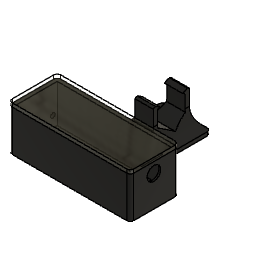
Sun_Flower_Step_Up_Support (Autodesk Fusion 360 design; units mm, degrees)
Autodesk Fusion 360 part; units mm, degrees
sketch "Sketch1" plane through (0, 0, 0) normal (0, 0, 1) x (1, 0, 0)
  line L0 (25, 9) -> (-25, 9)
  line L1 (-25, 9) -> (-25, -9)
  line L2 (-25, -9) -> (25, -9)
  line L3 (25, -9) -> (25, 9)
  line L4 (25, 9) -> (-25, -9) construction
  line L5 (-25, 9) -> (25, -9) construction
  line L6 (-26.6, -10.6) -> (26.6, -10.6)
  line L7 (26.6, -10.6) -> (26.6, 10.6)
  line L8 (26.6, 10.6) -> (-26.6, 10.6)
  line L9 (-26.6, 10.6) -> (-26.6, -10.6)
  dimension "d1" = 50
  dimension "d2" = 18
  dimension "d5" = 1.6
  constraint horizontal L0
  constraint perpendicular L0 L1
  constraint parallel L0 L2
  constraint parallel L1 L3
  constraint coincident L4 origin
  constraint coincident L5 origin
  measures "d1" distance of L1.end L2.end
  measures "d2" distance of L0.end L1.end
extrude "Extrude1" add sketch "Sketch1" along normal blind 1.2 contours L0 L1 L2 L3 makes body 1
extrude "Extrude2" add sketch "Sketch1" along normal blind 18 bodies 1
sketch "Sketch6" plane through (25, 0, 0) normal (-1, 0, 0) x (0, -1, 0)
  line L0 (-9, 1.2) -> (9, 1.2)
  line L1 (9, 1.2) -> (9, 18)
  line L2 (9, 18) -> (-9, 18)
  line L3 (-9, 18) -> (-9, 1.2)
  line L4 (-4.3225, 18) -> (4.8375, 18)
  line L5 (4.8375, 18) -> (4.8375, 6.4)
  line L6 (4.8375, 6.4) -> (-4.3225, 6.4)
  line L7 (-4.3225, 6.4) -> (-4.3225, 18)
  line L8 (4.6375, 6.6) -> (-4.1225, 6.6)
  line L9 (-4.1225, 6.6) -> (-4.1225, 17.8)
  line L10 (-4.1225, 17.8) -> (4.6375, 17.8)
  line L11 (4.6375, 17.8) -> (4.6375, 6.6)
  point P0 (-4.3225, 18)
  point P1 (4.8375, 6.4)
  dimension "d27" = 0.2
  dimension "d62" = 11.6
  constraint horizontal L4
  constraint vertical L5
  constraint horizontal L6
  constraint vertical L7
  constraint coincident P1 L5.end
  constraint coincident P0 L4.start
  constraint coincident L2 L4.end
  measures "d62" distance of L4 L6
extrude "Extrude3" cut sketch "Sketch6" against normal blind 0.8 contours L2 L4 L5 L6 L7 | L8 L9 L10 L11 bodies 1
sketch "Sketch3" plane through (26.6, 0, 0) normal (1, 0, 0) x (0, 1, 0)
  line L0 (-10.6, 0) -> (10.6, 0)
  line L1 (10.6, 0) -> (10.6, 18)
  line L2 (10.6, 18) -> (-10.6, 18)
  line L3 (-10.6, 18) -> (-10.6, 0)
  circle A0 centre (-0.2575, 13.52) radius 3
  dimension "d63" = 4.48
  measures "d63" distance of L2 A0.centre
extrude "Extrude4" cut sketch "Sketch3" against normal blind 2 contours A0 bodies 1
sketch "Sketch4" plane through (-26.6, 0, 0) normal (-1, 0, 0) x (0, -1, 0)
  line L0 (-10.6, 0) -> (10.6, 0)
  line L1 (10.6, 0) -> (10.6, 18)
  line L2 (10.6, 18) -> (-10.6, 18)
  line L3 (-10.6, 18) -> (-10.6, 0)
  circle A0 centre (-7.1, 6) radius 1
  dimension "d13" = 2
  dimension "d14" = 6
  dimension "d15" = 3.5
  measures "d13" diameter of A0
  measures "d14" distance of L0 A0.centre
  measures "d15" distance of L3 A0.centre
extrude "Extrude5" cut sketch "Sketch4" against normal blind 1.6 contours A0 bodies 1
mirror "Mirror1" about plane through (0, 0, 0) normal (0, 1, 0) of "Extrude5"
sketch "Sketch5" plane through (0, 0, 18) normal (0, 0, 1) x (-1, 0, 0)
  line L0 (26.6, -10.6) -> (26.6, 10.6)
  line L1 (26.6, 10.6) -> (-26.6, 10.6)
  line L2 (-26.6, 10.6) -> (-26.6, -10.6)
  line L3 (-26.6, -10.6) -> (26.6, -10.6)
  line L4 (-25, 4.8375) -> (-25, 9)
  line L5 (-25, 9) -> (25, 9)
  line L6 (25, 9) -> (25, -9)
  line L7 (25, -9) -> (-25, -9)
  line L8 (26.6, -10.6) -> (-26.6, -10.6)
  line L9 (-26.6, -10.6) -> (-26.6, 10.6)
  line L10 (-26.6, 10.6) -> (26.6, 10.6)
  line L11 (26.6, 10.6) -> (26.6, -10.6)
  line L12 (-25.8, -4.3225) -> (-25.8, 4.8375)
  line L13 (-25.8, 4.8375) -> (-25, 4.8375)
  line L14 (-25, -9) -> (-25, -4.3225)
  line L15 (-25, -4.3225) -> (-25.8, -4.3225)
  line L16 (26.6, -10.6) -> (26.6, 10.6)
  line L17 (26.6, 10.6) -> (-26.6, 10.6)
  line L18 (-26.6, 10.6) -> (-26.6, -10.6)
  line L19 (-26.6, -10.6) -> (26.6, -10.6)
  line L20 (-25, -4.3225) -> (-25.8, -4.3225)
  line L21 (-25.8, -4.3225) -> (-25.8, 4.8375)
  line L22 (-25.8, 4.8375) -> (-25, 4.8375)
  line L23 (-25, 4.8375) -> (-25, 9)
  line L24 (-25, 9) -> (25, 9)
  line L25 (25, 9) -> (25, -9)
  line L26 (25, -9) -> (-25, -9)
  line L27 (-25, -9) -> (-25, -4.3225)
  constraint horizontal L8
  constraint vertical L9
  constraint horizontal L10
  constraint vertical L11
  constraint coincident L1.end L2.start
  constraint coincident L0.start L3.end
extrude "Extrude7" add sketch "Sketch5" along normal blind 1.6 separate body contours L0 L1 L2 L3 L8 L9 L10 L11 L16 L17 L18 L19 | L4 L5 L6 L7 L12 L13 L14 L15 L20 L21 L22 L23 L24 L25 L26 L27 makes body 2
fillet "Fillet1" radius 1.5 8 edges at (-26.6, -10.6, 9) (-26.6, 10.6, 9) (26.6, 10.6, 9) (26.6, -10.6, 9) (-26.6, -10.6, 18.8) (-26.6, 10.6, 18.8) (26.6, 10.6, 18.8) (26.6, -10.6, 18.8) on bodies 1 2
move_body "Move4" bodies 2 to x (1, 0, 0) y (0, 1, 0) z (0, 0, 1) at (0, 0, -0.15)
sketch "Sketch9" plane through (0, 0, 1.2) normal (0, 0, 1) x (-1, 0, 0)
  line L0 (-25, 9) -> (-25, -9)
  line L1 (-25, -9) -> (25, -9)
  line L2 (25, -9) -> (25, 9)
  line L3 (25, 9) -> (-25, 9)
  circle A0 centre (23.5, 7.15) radius 1
  circle A1 centre (-10, 7.15) radius 1
  dimension "d49" = 2
  dimension "d50" = 1.5
  dimension "d51" = 1.85
  dimension "d56" = 2
  dimension "d57" = 15
  dimension "d58" = 1.85
  measures "d49" diameter of A0
  measures "d50" distance of L2 A0.centre
  measures "d51" distance of L3 A0.centre
  measures "d56" diameter of A1
  measures "d57" distance of L0 A1.centre
  measures "d58" distance of L3 A1.centre
extrude "Extrude12" cut sketch "Sketch9" against normal blind 1.2 contours A0 | A1 bodies 1
mirror "Mirror2" about plane through (0, 0, 0) normal (0, 1, 0) of "Extrude12"
move_body "Move1" bodies 2 to x (1, 0, 0) y (0, 1, 0) z (0, 0, 1) at (0, 0, 0.0101)
move_body "Move5" bodies 2 to x (1, 0, 0) y (0, 1, 0) z (0, 0, 1) at (0, 0, 0.15)
sketch "Sketch7" plane through (0, 0, 0) normal (0, 0, 1) x (1, 0, 0)
  line L0 (10.6, -10.6) -> (-10.6, -10.6)
  line L1 (-10.6, -10.6) -> (-10.6, 10.6)
  line L2 (-10.6, 10.6) -> (10.6, 10.6)
  line L3 (10.6, 10.6) -> (10.6, -10.6)
  line L4 (10.6, -10.6) -> (-10.6, 10.6) construction
  line L5 (-10.6, -10.6) -> (10.6, 10.6) construction
  dimension "d28" = 21.2
  dimension "d29" = 21.2
  constraint horizontal L0
  constraint perpendicular L0 L1
  constraint parallel L0 L2
  constraint parallel L1 L3
  constraint coincident L4 origin
  constraint coincident L5 origin
  measures "d28" distance of L1.end L2.end
  measures "d29" distance of L0.end L1.end
extrude "Extrude8" add sketch "Sketch7" along normal blind 1.6 separate body makes body 3
sketch "Sketch8" plane through (0, 0, 0) normal (1, 0, 0) x (0, 1, 0)
  line L0 (0, 4.0249) -> (5.8639, 7.4104)
  line L1 (5.8639, 7.4104) -> (5.8639, 14.1814)
  line L2 (5.8639, 14.1814) -> (0, 17.5669)
  line L3 (0, 17.5669) -> (-5.8639, 14.1814)
  line L4 (-5.8639, 14.1814) -> (-5.8639, 7.4104)
  line L5 (-5.8639, 7.4104) -> (0, 4.0249)
  line L6 (-7.9639, 15.3938) -> (-7.9639, 6.1979)
  line L7 (-7.9639, 6.1979) -> (0, 1.6)
  line L8 (0, 1.6) -> (7.9639, 6.1979)
  line L9 (7.9639, 6.1979) -> (7.9639, 15.3938)
  line L10 (7.9639, 15.3938) -> (0, 19.9917)
  line L11 (0, 19.9917) -> (-7.9639, 15.3938)
  line L12 (-6.0139, 14.268) -> (-6.0139, 7.3238)
  line L13 (-6.0139, 7.3238) -> (0, 3.8517)
  line L14 (0, 3.8517) -> (6.0139, 7.3238)
  line L15 (6.0139, 7.3238) -> (6.0139, 14.268)
  line L16 (6.0139, 14.268) -> (0, 17.7401)
  line L17 (0, 17.7401) -> (-6.0139, 14.268)
  line L18 (-7.9639, 6.1979) -> (-7.9639, 1.6)
  line L19 (-7.9639, 1.6) -> (0, 1.6)
  line L20 (7.9639, 6.1979) -> (7.9639, 1.6)
  line L21 (7.9639, 1.6) -> (0, 1.6)
  line L22 (-7.9639, 15.3938) -> (-6.0139, 14.268)
  line L23 (6.0139, 14.268) -> (7.9639, 15.3938)
  line L24 (-6.9639, 15.9712) -> (-5.0139, 14.8453)
  line L25 (6.9639, 15.9712) -> (5.0139, 14.8453)
  line L26 (-7.2139, 14.9608) -> (-7.2139, 6.6309)
  line L27 (-7.2139, 6.6309) -> (0, 2.466)
  line L28 (0, 2.466) -> (7.2139, 6.6309)
  line L29 (7.2139, 6.6309) -> (7.2139, 14.9608)
  line L30 (7.2139, 14.9608) -> (0, 19.1257)
  line L31 (0, 19.1257) -> (-7.2139, 14.9608)
  line L32 (-7.2139, 6.6309) -> (-7.2139, 1.6)
  line L33 (7.2139, 6.6309) -> (7.2139, 1.6)
  point P0 (0, 10.7959)
  dimension "d32" = 6.771
  dimension "d33" = 2.1
  dimension "d34" = 0.15
  dimension "d35" = 1
  dimension "d36" = 1
  dimension "d59" = 1.35
  constraint coincident L7.end
  constraint parallel L6 L18
  constraint perpendicular L18 L19
  constraint perpendicular L19 L20
  constraint perpendicular L20 L21
  constraint coincident L11 L24.start
  constraint coincident L17 L24.end
  constraint parallel L22 L24
  constraint coincident L10 L25.start
  constraint coincident L16 L25.end
  constraint parallel L11 L25
  constraint coincident L19 L32.end
  constraint perpendicular L19 L32
  constraint coincident L21 L33.end
  constraint perpendicular L21 L33
  measures "d32" distance of L0.start P0
  measures "d35" distance of L22 L24
  measures "d36" distance of L23 L25
extrude "Extrude9" add sketch "Sketch8" along normal blind 4 separate body contours L6 L7 L22 L26 L32 | L11 L22 L24 L31 | L7 L18 L19 L32 | L17 L22 L24 L31 | L12 L13 L14 L15 L22 L23 L26 L27 L28 L29 | L7 L8 L27 L28 L32 L33 | L7 L19 L32 | L8 L21 L33 | L10 L23 L25 L30 | L8 L9 L23 L29 L33 | L8 L20 L21 L33 | L16 L23 L25 L30 makes body 4
extrude "Extrude10" add 1 faces at (0, 4.4092, 4.2585) along direction (-1, 0, 0) blind 4 on bodies 4 bodies 3 4
fillet "Fillet2" radius 7 4 edges at (-4, 0, 1.6) (4, 0, 1.6) (0, 7.9639, 1.6) (0, -7.9639, 1.6) on bodies 3
fillet "Fillet2" radius 1.5 4 edges at (-10.6, 10.6, 0.8) (10.6, 10.6, 0.8) (-10.6, -10.6, 0.8) (10.6, -10.6, 0.8) on bodies 3
move_body "Move2" bodies 1 2 to x (1, 0, 0) y (0, 1, 0) z (0, 0, 1) at (0, -15, 0)
move_body "Move3" bodies 3 to x (1, 0, 0) y (0, 1, 0) z (0, 0, 1) at (0, 15, 0)
copy_body "CutPasteBodies1" bodies 1 2 removing the originals makes body 5 makes body 6 in component "Case"
copy_body "CutPasteBodies1'" bodies 3 removing the originals makes body 7 in component "Support"
component "Case" placed x (1, 0, 0) y (0, 1, 0) z (0, 0, 1) at (0, 0, 0)
component "Support" placed x (1, 0, 0) y (0, 1, 0) z (0, 0, 1) at (0, 0, 0)
equation "d36 = d35"
equation "d63 = 1.48 mm + 3 mm"
named bodies: "Case", "Cap", "Support"
